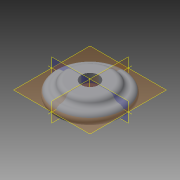
# Autodesk Inventor part: LenkStangeSicherung
Saved by Autodesk Inventor 2015 (Build 190159000, 159)
## iProperties
Created: 2018-11-02
Part Number: LenkStangeSicherung
Material: Generisch
Document SubType Name: Modeling
Designer: Boris
Density: 1 g/cm^3
Appearance: Vorgabe
Author: Boris
Autodesk Inventor part; units mm, degrees
sketch "Skizze1" plane through (0, 0, 0) normal (0, 0, 1) x (1, 0, 0)
  circle A0 centre (0, 0) radius 6
  dimension "d0" = 12
  constraints: 1 centre point, 1 coincident
  measures "d0" diameter of A0
extrude "Extrusion1" add sketch "Skizze1" along normal mid plane 3
sketch "Skizze2" plane through (0, 0, 1.5) normal (0, 0, 1) x (1, 0, 0)
  circle A0 centre (0, 0) radius 6 projected
  circle A1 centre (0, 0) radius 4
  dimension "d3" = 8
  constraints: 1 centre point, 1 coincident
  measures "d3" diameter of A1
extrude "Extrusion2" cut sketch "Skizze2" against normal blind 1
sketch "Skizze3" plane through (0, 0, 1.5) normal (0, 0, 1) x (1, 0, 0)
  circle A0 centre (0, 0) radius 1.5
  dimension "d6" = 3
  constraints: 1 centre point, 1 coincident
  measures "d6" diameter of A0
extrude "Extrusion3" cut sketch "Skizze3" against normal blind 5
sketch "Skizze4" plane through (0, 0, -1.5) normal (0, 0, -1) x (-1, 0, 0)
  circle A0 centre (0, 0) radius 1.5 projected
  circle A1 centre (0, 0) radius 3
  dimension "d9" = 1.5
  constraints: 1 centre point
  measures "d9" radial gap between concentric circles of A0 A1
extrude "Extrusion4" cut sketch "Skizze4" against normal blind 1.5
fillet "Rundung1" radius 2 1 edges at (3, 0, 0)
fillet "Rundung2" radius 1 2 edges at (-4, 0, 0.5) (-4, 0, 1.5)
fillet "Rundung3" radius 1 1 edges at (3, 0, -1.5)
fillet "Rundung4" radius 1 2 edges at (-6, 0, -1.5) (-6, 0, 0.5)
